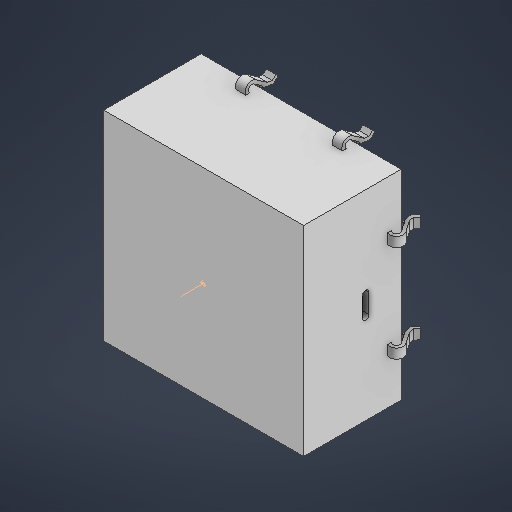
# Autodesk Inventor part: Top_part
Saved by Autodesk Inventor 2027 (Build 310192000, 192)
## iProperties
Created: 2026-04-01
Part Number: Top_part
Material: Generic
Document SubType Name: Modeling
Designer: thomas
Density: 1 g/cm^3
Appearance: Default
Author: thomas
Autodesk Inventor part; units mm, degrees
ref_plane "YZ Plane" through (0, 0, 0) normal (1, 0, 0) x (0, 1, 0)
ref_plane "XZ Plane" through (0, 0, 0) normal (0, 1, 0) x (-1, 0, 0)
ref_plane "XY Plane" through (0, 0, 0) normal (0, 0, 1) x (1, 0, 0)
ref_plane "Work Plane13" through (32.2002, -87.6795, 34.9894) normal (0, 0, 1) x (1, 0, 0)
sketch "Sketch8" plane through (32.2002, -87.6795, 34.9894) normal (0, 0, 1) x (1, 0, 0)
  line L0 (62, -62) -> (-62, -62)
  line L1 (-62, -62) -> (-62, 62)
  line L2 (-62, 62) -> (62, 62)
  line L3 (62, 62) -> (62, -62)
  line L4 (62, -62) -> (-62, 62) construction
  line L5 (-62, -62) -> (62, 62) construction
  line L6 (56, -56) -> (-56, -56)
  line L7 (-56, -56) -> (-56, 56)
  line L8 (-56, 56) -> (56, 56)
  line L9 (56, 56) -> (56, -56)
  line L10 (56, -56) -> (-56, 56) construction
  line L11 (-56, -56) -> (56, 56) construction
  point P0 (-32.2002, 87.6795)
  point P1 (0, 0)
  point P2 (0, 0)
  constraints: 24 end point, 5 midpoint, 5 parallel, 2 perpendicular, 1 horizontal
extrude "Extrusion1" add sketch "Sketch8" along normal blind 55
sketch "Sketch14" plane through (32.2002, -87.6795, 89.9894) normal (0, 0, 1) x (1, 0, 0)
  line L0 (-62, -62) -> (62, -62) projected
  line L1 (62, 62) -> (-62, 62) projected
  line L2 (62, -62) -> (-62, -62)
  line L3 (-62, -62) -> (-62, 62)
  line L4 (-62, 62) -> (62, 62)
  line L5 (62, 62) -> (62, -62)
  constraints: 8 end point, 2 parallel, 1 horizontal, 1 perpendicular
extrude "Extrusion2" add sketch "Sketch14" along normal blind 5.5
ref_plane "Work Plane8" through (32.2002, -149.6795, 34.9894) normal (-1, 0, 0) x (0, 0, 1)
ref_plane "Work Plane9" through (1.2002, -149.6795, 34.9894) normal (-1, 0, 0) x (0, 0, 1)
sketch "Sketch17" plane through (1.2002, -149.6795, 34.9894) normal (-1, 0, 0) x (0, 0, 1)
  line L0 (0, 0) -> (2.5493, -4.1672) construction
  arc A0 (2.5493, -4.1672) -> (6.5801, 0.8328) centre (4.5647, -1.6672) ccw
  line L1 (6.5801, 0.8328) -> (3.4598, 1.8328)
  line L2 (-19.9665, 21.2414) -> (-11.1433, 19.7708) construction
  line L3 (2.5493, -4.1672) -> (-4.6608, 0.8328)
  line L4 (-4.6608, 0.8328) -> (-8.4211, 1.4595)
  line L5 (-8.4211, 1.4595) -> (-11, -1)
  point P0 (-34.9894, 149.6795)
  constraints: 12 end point, 2 point on circle, 1 centre point
ref_plane "Work Plane15" through (1.2002, -150.6795, 23.9894) normal (0, -0.6901647, -0.7236523) x (1, 0, 0)
sketch "Sketch24" plane through (1.2002, -150.6795, 23.9894) normal (0, -0.6901647, -0.7236523) x (1, 0, 0)
  line L0 (3, -1) -> (-3, -1)
  line L1 (-3, -1) -> (-3, 1)
  line L2 (-3, 1) -> (3, 1)
  line L3 (3, 1) -> (3, -1)
  line L4 (3, -1) -> (-3, 1) construction
  line L5 (-3, -1) -> (3, 1) construction
  point P0 (-1.2002, -125.5962)
  point P1 (0, 0)
  point P2 (0, 0)
  constraints: 12 end point, 2 midpoint, 2 parallel, 1 coincident, 1 horizontal, 1 perpendicular
sweep "Sweep4" add profiles "Sketch24" path "Sketch17"
ref_plane "Work Plane16" through (-1.7998, -147.8972, 30.7143) normal (0, 0.164399, -0.9863939) x (-1, 0, 0)
sketch "Sketch26" plane through (-1.7998, -147.8972, 30.7143) normal (0, 0.164399, -0.9863939) x (-1, 0, 0)
  line L0 (0, 0) -> (-5.9818, 0)
  line L1 (-5.9818, 0) -> (-5.9818, -2.1725)
  line L2 (-5.9818, -2.1725) -> (0, -2.1725)
  line L3 (0, -2.1725) -> (0, 0)
  point P0 (-1.7998, 140.8355)
  constraints: 8 end point, 2 parallel, 1 horizontal, 1 perpendicular
extrude "Extrusion4" add sketch "Sketch26" against normal blind 2.5
sketch "Sketch25" plane through (-29.7998, -149.6795, 34.9894) normal (0, -1, 0) x (1, 0, 0)
  line L0 (56, 24) -> (68, 24)
  line L1 (68, 24) -> (68, 20)
  line L2 (68, 20) -> (56, 20)
  line L3 (56, 20) -> (56, 24)
  line L4 (56, 24) -> (68, 20) construction
  line L5 (68, 24) -> (56, 20) construction
  circle A0 centre (56, 22) radius 2
  circle A1 centre (68, 22) radius 2
  line L6 (62, -129.3185) -> (62, 92.1364) projected
  point P0 (29.7998, -34.9894)
  point P1 (62, 22)
  point P2 (56, 24)
  point P3 (56, 20)
  point P4 (68, 20)
  constraints: 12 end point, 4 midpoint, 2 centre point, 2 parallel, 1 horizontal, 1 perpendicular, 1 point on line
extrude "Extrusion3" cut sketch "Sketch25" against normal blind 6
pattern_circular "Circular Pattern4" count 4 over 360 about axis through (32.2002, -87.6795, 95.4894) along (0, 0, 1) of "Extrusion3"
sketch "Sketch27" plane through (-29.7998, -149.6795, 34.9894) normal (-1, 0, 0) x (0, 0, 1)
  line L0 (0, 124) -> (60.5, 124) projected
  line L1 (30.5, 124) -> (26.5, 124)
  line L2 (26.5, 124) -> (26.5, 69)
  line L3 (26.5, 69) -> (30.5, 69)
  line L4 (30.5, 69) -> (30.5, 124)
  line L5 (60.5, 124) -> (60.5, 0) projected
  line L6 (26.5, 69) -> (13.7708, 124)
  line L7 (26.5, 124) -> (13.7708, 124)
  point P0 (-34.9894, 149.6795)
  dimension "d51" = 4
  dimension "d52" = 30
  dimension "d53" = 55
  constraints: 12 end point, 2 parallel, 2 point on line, 1 collinear, 1 horizontal, 1 perpendicular
  measures "d51" distance of L3.end L2.end
  measures "d52" distance between parallel lines of L5 L4
  measures "d53" distance between parallel lines of L0 L3
extrude "Extrusion5" add sketch "Sketch27" against normal blind 75
pattern_linear "Rectangular Pattern7" count 2 spacing 60 along (1, 0, 0) of "Sweep4", "Extrusion4"
pattern_circular "Circular Pattern6" count 4 over 360 about axis through (32.2002, -87.6795, 95.4894) along (0, 0, 1) of "Sweep4", "Extrusion4", "Rectangular Pattern7"
body "Solid1"
body "Solid5"
